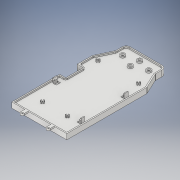
# Autodesk Inventor part: Display_Plate
Saved by Autodesk Inventor 2018 (Build 220112000, 112)
## iProperties
Created: 2019-05-28
Part Number: Display_Plate
Material: ABS Plastic
Document SubType Name: Modeling
Designer: Ash
Density: 1.06 g/cm^3
Appearance: Smooth - White
Author: Ash
Autodesk Inventor part; units mm, degrees
ref_plane "YZ Plane" through (0, 0, 0) normal (1, 0, 0) x (0, 1, 0)
ref_plane "XZ Plane" through (0, 0, 0) normal (0, 1, 0) x (-1, 0, 0)
ref_plane "XY Plane" through (0, 0, 0) normal (0, 0, 1) x (1, 0, 0)
sketch "Sketch1" plane through (0, 0, 0) normal (0, 1, 0) x (-1, 0, 0)
  line L0 (-80.01, -1.2579) -> (-80.01, -117.3941)
  line L1 (-80.01, -118.0979) -> (0, -118.0979) construction
  line L2 (0, -117.3941) -> (0, -96.3809)
  line L3 (-79.7125, -118.7359) -> (-69.5125, -140.61)
  line L4 (-80.01, -118.0979) -> (-55.8746, -118.0979) construction
  line L5 (-0.2975, -118.7359) -> (-10.4975, -140.61)
  line L6 (0, -118.0979) -> (24.1354, -118.0979) construction
  line L7 (-10.795, -141.2479) -> (-69.215, -141.2479) construction
  line L8 (-69.215, -141.9518) -> (-69.215, -150.6459)
  line L9 (-62.865, -156.9959) -> (-17.145, -156.9959)
  line L10 (-10.795, -150.6459) -> (-10.795, -141.9518)
  arc A0 (-0.2975, -118.7359) -> (0, -117.3941) centre (-3.175, -117.3941) ccw
  arc A1 (-80.01, -117.3941) -> (-79.7125, -118.7359) centre (-76.835, -117.3941) ccw
  arc A2 (-69.215, -150.6459) -> (-62.865, -156.9959) centre (-62.865, -150.6459) ccw
  arc A3 (-17.145, -156.9959) -> (-10.795, -150.6459) centre (-17.145, -150.6459) ccw
  arc A4 (-10.4975, -140.61) -> (-10.795, -141.9518) centre (-7.62, -141.9518) ccw
  arc A5 (-69.215, -141.9518) -> (-69.5125, -140.61) centre (-72.39, -141.9518) ccw
  line L11 (0, -96.3809) -> (-8.763, -96.3809)
  line L12 (-8.763, -96.3809) -> (-8.763, -70.9809)
  line L13 (-8.763, -70.9809) -> (0, -70.9809)
  line L14 (-80.01, -1.2579) -> (0, -1.2579)
  line L15 (0, -70.9809) -> (0, -1.2579)
  point P0 (0, 0)
  point P1 (-69.215, -156.9959)
  dimension "d0" = 80.01
  dimension "d1" = 116.84
  dimension "d3" = 65
  dimension "d4" = 115
  dimension "d5" = 58.42
  dimension "d6" = 15.748
  dimension "d7" = 3.175
  dimension "d8" = 6.35
  dimension "d9" = 3.175
  dimension "d45" = 8.763
  dimension "d46" = 25.4
  dimension "d47" = 21.717
  constraints: 32 end point, 12 point on circle, 12 point on line, 12 tangent, 6 centre point, 5 horizontal, 4 parallel, 4 perpendicular, 3 equal radius, 2 equal length, 1 horizontal alignment, 1 vertical
  measures "d0" distance of L1.end L1.start
  measures "d1" distance of L0.start L1.start
  measures "d3" angle of L3 L4
  measures "d4" angle of L5 L6
  measures "d5" distance of point (-69.215, -141.248) L7.start
  measures "d6" distance of point (-69.215, -156.996) L7.end
  measures "d7" radius of A0
  measures "d8" radius of A2
  measures "d9" radius of A4
  measures "d45" distance of L2.end L11.end
  measures "d46" distance of L11.end L12.end
  measures "d47" distance from line of L1.end L11
extrude "Extrusion1" add sketch "Sketch1" along normal blind 3.81
shell "Shell1" thickness 1.778 removed faces 1 at (56.261, 3.81, -63.211)
sketch "Sketch2" plane through (1.778, 1.778, -1.778) normal (0, 1, 0) x (1, 0, 0)
  arc A0 (65.659, 140.1738) -> (66.1231, 138.0805) centre (70.612, 140.1738) ccw projected
  line L0 (65.7764, 139.1017) -> (60.579, 139.1017)
  line L1 (65.659, 148.8679) -> (65.659, 140.1738) projected
  line L2 (65.659, 140.6257) -> (60.579, 140.6257)
  line L3 (76.454, 115.6161) -> (76.454, 1.2579) projected
  arc A1 (76.454, 115.6161) -> (76.3231, 116.2065) centre (75.057, 115.6161) ccw projected
  line L4 (66.1231, 138.0805) -> (76.3231, 116.2065) projected
  arc A2 (65.659, 140.1738) -> (66.1231, 138.0805) centre (70.612, 140.1738) ccw projected
  line L5 (65.659, 148.8679) -> (65.659, 140.1738) projected
  arc A3 (65.659, 148.8679) -> (61.087, 153.4399) centre (61.087, 148.8679) ccw construction
  line L6 (15.367, 153.4399) -> (61.087, 153.4399) construction
  arc A4 (15.367, 153.4399) -> (10.795, 148.8679) centre (15.367, 148.8679) ccw construction
  line L7 (10.795, 140.1738) -> (10.795, 148.8679) projected
  arc A5 (10.3309, 138.0805) -> (10.795, 140.1738) centre (5.842, 140.1738) ccw projected
  line L8 (0.1309, 116.2065) -> (10.3309, 138.0805) construction
  arc A6 (0.1309, 116.2065) -> (0, 115.6161) centre (1.397, 115.6161) ccw projected
  line L9 (0, 96.3809) -> (0, 115.6161) projected
  circle A7 centre (57.2357, 139.8637) radius 1.905
  circle A8 centre (57.2357, 139.8637) radius 3.429
  line L10 (65.7764, 139.8637) -> (47.2298, 139.8637) construction
  line L11 (15.367, 153.4399) -> (61.087, 153.4399) construction
  line L12 (38.227, 153.4399) -> (38.227, -24.5514) construction
  line L13 (57.2357, 139.8637) -> (57.2357, 153.4399) construction
  line L14 (56.4737, 143.207) -> (56.4737, 153.4399)
  line L15 (57.9977, 143.2111) -> (57.9977, 153.4399)
  line L16 (57.2357, 139.8637) -> (38.227, 145.4827) construction
  line L17 (57.2357, 139.8637) -> (38.227, 132.0207) construction
  circle A9 centre (38.227, 132.0207) radius 1.905
  circle A10 centre (38.227, 145.4827) radius 1.905
  circle A11 centre (38.227, 132.0207) radius 3.429
  circle A12 centre (38.227, 145.4827) radius 3.429
  line L18 (41.6491, 145.2657) -> (54.2456, 141.5422)
  line L19 (59.5161, 139.9683) -> (54.4955, 137.8025) construction
  line L20 (41.2171, 143.8042) -> (53.8136, 140.0807)
  line L21 (54.9501, 139.7414) -> (53.8727, 139.1943) construction
  line L22 (53.8136, 140.0807) -> (54.9501, 139.7414) construction
  line L23 (53.8727, 139.1943) -> (41.0645, 133.946)
  line L24 (54.2456, 141.5422) -> (59.5161, 139.9683) construction
  line L25 (54.4955, 137.8025) -> (41.6186, 132.5261)
  line L26 (10.6776, 139.1017) -> (15.875, 139.1017)
  line L27 (10.795, 140.6257) -> (15.875, 140.6257)
  circle A13 centre (19.2183, 139.8637) radius 1.905
  circle A14 centre (19.2183, 139.8637) radius 3.429
  line L28 (19.9803, 143.207) -> (19.9803, 153.4399)
  line L29 (18.4563, 143.2111) -> (18.4563, 153.4399)
  line L30 (34.8049, 145.2657) -> (22.2084, 141.5422)
  line L31 (35.2369, 143.8042) -> (22.6404, 140.0807)
  line L32 (22.5813, 139.1943) -> (35.3895, 133.946)
  line L33 (21.9585, 137.8025) -> (34.8354, 132.5261)
  line L34 (34.8354, 132.5261) -> (21.9585, 137.8025)
  line L35 (22.5813, 139.1943) -> (35.3895, 133.946)
  circle A15 centre (38.227, 132.0207) radius 3.429
  circle A16 centre (38.227, 145.4827) radius 3.429
  circle A17 centre (19.2183, 139.8637) radius 3.429
  line L36 (15.367, 153.4399) -> (61.087, 153.4399) projected
  line L37 (8.763, 96.3809) -> (0, 96.3809) projected
  line L38 (8.763, 67.4249) -> (8.763, 96.3809) projected
  line L39 (0, 67.4249) -> (8.763, 67.4249) projected
  line L40 (0, 1.2579) -> (0, 67.4249) projected
  line L41 (76.454, 1.2579) -> (0, 1.2579) projected
  point P0 (-1.778, -1.778)
  dimension "d13" = 1.524
  dimension "d14" = 5.08
  dimension "d15" = 3.81
  dimension "d16" = 1.524
  dimension "d17" = 0.762
  dimension "d20" = 1.524
  dimension "d21" = 0.762
  dimension "d22" = 13.462
  dimension "d23" = 3.81
  dimension "d24" = 3.81
  dimension "d25" = 1.524
  dimension "d26" = 1.524
  dimension "d27" = 0.762
  dimension "d28" = 0.762
  dimension "d30" = 1.524
  constraints: 54 end point, 17 symmetric about line, 7 centre point, 7 point on line, 6 point on circle, 5 coincident, 4 parallel, 2 horizontal, 2 vertical, 1 concentric, 1 midpoint, 1 perpendicular, 28 other
  measures "d13" distance between parallel lines of L0 L2
  measures "d14" distance of L2.start L2.end
  measures "d15" diameter of A7
  measures "d17" distance between parallel lines of L0 L10
  measures "d20" distance between parallel lines of L15 L14
  measures "d21" distance between parallel lines of L13 L14
  measures "d22" distance of L16.end L17.end
  measures "d23" diameter of A9
  measures "d24" diameter of A10
  measures "d25" radial gap between concentric circles of A9 A11
  measures "d26" radial gap between concentric circles of A10 A12
  measures "d27" distance between parallel lines of L16 L18
  measures "d28" distance between parallel lines of L16 L20
  measures "d30" distance between parallel lines of L25 L23
sketch "Sketch3" plane through (1.778, 1.778, -1.778) normal (0, 1, 0) x (1, 0, 0)
  circle A0 centre (19.2183, 139.7488) radius 1.905 projected
  circle A1 centre (19.2183, 139.7488) radius 3.429 projected
  circle A2 centre (38.227, 145.4827) radius 1.905 projected
  circle A3 centre (38.227, 145.4827) radius 3.429 projected
  circle A4 centre (38.227, 132.0207) radius 1.905 projected
  circle A5 centre (38.227, 132.0207) radius 3.429 projected
  circle A6 centre (57.2357, 139.7488) radius 1.905 projected
  circle A7 centre (57.2357, 139.7488) radius 3.429 projected
  arc A8 (60.579, 140.5108) -> (60.579, 140.5108) centre (57.2357, 139.7488) ccw projected
  line L0 (58.0015, 143.0912) -> (58.0015, 153.325)
  line L1 (15.367, 153.4399) -> (61.087, 153.4399) projected
  line L2 (56.4718, 153.325) -> (56.4718, 143.0916)
  line L3 (65.659, 148.8679) -> (65.659, 140.1738) projected
  arc A9 (65.659, 148.8679) -> (61.087, 153.4399) centre (61.087, 148.8679) ccw projected
  line L4 (15.367, 153.4399) -> (61.087, 153.4399) projected
  arc A10 (15.367, 153.4399) -> (10.795, 148.8679) centre (15.367, 148.8679) ccw projected
  line L5 (10.795, 140.1738) -> (10.795, 148.8679) projected
  arc A11 (10.3309, 138.0805) -> (10.795, 140.1738) centre (5.842, 140.1738) ccw projected
  line L6 (0.1309, 116.2065) -> (10.3309, 138.0805) projected
  arc A12 (0.1309, 116.2065) -> (0, 115.6161) centre (1.397, 115.6161) ccw projected
  line L7 (0, 96.3809) -> (0, 115.6161) projected
  line L8 (76.454, 115.6161) -> (76.454, 1.2579) projected
  arc A13 (76.454, 115.6161) -> (76.3231, 116.2065) centre (75.057, 115.6161) ccw projected
  line L9 (66.1231, 138.0805) -> (76.3231, 116.2065) projected
  arc A14 (65.659, 140.1738) -> (66.1231, 138.0805) centre (70.612, 140.1738) ccw projected
  line L10 (18.4767, 153.4399) -> (18.4767, 143.2116)
  circle A15 centre (19.2183, 139.7488) radius 3.429 projected
  line L11 (19.9598, 143.0967) -> (19.9598, 153.4399)
  line L12 (22.199, 141.4439) -> (34.8061, 145.2467)
  arc A16 (41.656, 145.4827) -> (41.656, 145.4827) centre (38.227, 145.4827) ccw projected
  line L13 (35.2463, 143.7877) -> (22.6391, 139.9848)
  line L14 (22.023, 137.7761) -> (34.8354, 132.5261)
  arc A17 (41.656, 132.0207) -> (41.656, 132.0207) centre (38.227, 132.0207) ccw projected
  line L15 (22.6008, 139.1863) -> (35.3895, 133.946)
  line L16 (15.875, 140.5108) -> (10.795, 140.5108)
  line L17 (10.795, 140.1738) -> (10.795, 148.8679) projected
  line L18 (15.875, 138.9868) -> (10.6776, 139.1017)
  line L19 (8.763, 96.3809) -> (0, 96.3809) projected
  line L20 (8.763, 67.4249) -> (8.763, 96.3809) projected
  line L21 (0, 67.4249) -> (8.763, 67.4249) projected
  line L22 (0, 1.2579) -> (0, 67.4249) projected
  line L23 (76.454, 1.2579) -> (0, 1.2579) projected
  point P0 (-1.778, -1.778)
  constraints: 20 end point, 7 point on circle, 3 point on line, 2 parallel, 2 vertical, 1 horizontal, 1 perpendicular, 9 other
sketch "Sketch5" plane through (1.778, 1.778, -1.778) normal (0, 1, 0) x (1, 0, 0)
  line L0 (0, 96.3809) -> (0, 115.6161) projected
  line L1 (0, 115.6161) -> (10.16, 115.6161) construction
  arc A0 (76.454, 115.6161) -> (76.3231, 116.2065) centre (75.057, 115.6161) ccw projected
  line L2 (76.3231, 116.2065) -> (66.1631, 116.2065) construction
  line L3 (-1.778, 69.2029) -> (-1.778, -1.778) projected
  line L4 (-1.778, 23.1379) -> (19.304, 23.1379) construction
  line L5 (-1.778, 23.1379) -> (19.304, 23.1379) construction
  line L6 (76.454, 23.1379) -> (55.372, 23.1379) construction
  line L7 (61.087, 155.2179) -> (15.367, 155.2179) projected
  line L8 (9.4963, 155.2179) -> (45.0563, 155.2179) construction
  line L9 (10.795, 140.5108) -> (22.6473, 140.5108) construction
  line L10 (10.16, 116.3781) -> (5.08, 116.3781)
  line L11 (5.08, 116.3781) -> (5.08, 114.8541)
  line L12 (5.08, 114.8541) -> (10.16, 114.8541)
  line L13 (10.16, 114.8541) -> (10.16, 116.3781)
  line L14 (6.858, 113.0761) -> (8.382, 113.0761)
  line L15 (8.382, 113.0761) -> (8.382, 118.1561)
  line L16 (8.382, 118.1561) -> (6.858, 118.1561)
  line L17 (6.858, 118.1561) -> (6.858, 113.0761)
  line L18 (6.858, 113.0761) -> (8.382, 118.1561) construction
  line L19 (8.382, 113.0761) -> (6.858, 118.1561) construction
  line L20 (7.62, 116.3781) -> (7.62, 114.8541) construction
  circle A1 centre (7.62, 115.6161) radius 0.889
  line L21 (68.7031, 115.4445) -> (63.6231, 115.4445)
  line L22 (63.6231, 115.4445) -> (63.6231, 116.9685)
  line L23 (63.6231, 116.9685) -> (68.7031, 116.9685)
  line L24 (68.7031, 116.9685) -> (68.7031, 115.4445)
  line L25 (65.4011, 113.6665) -> (66.9251, 113.6665)
  line L26 (66.9251, 113.6665) -> (66.9251, 118.7465)
  line L27 (66.9251, 118.7465) -> (65.4011, 118.7465)
  line L28 (65.4011, 118.7465) -> (65.4011, 113.6665)
  line L29 (65.4011, 113.6665) -> (66.9251, 118.7465) construction
  line L30 (66.9251, 113.6665) -> (65.4011, 118.7465) construction
  line L31 (66.1631, 115.4445) -> (66.1631, 116.9685) construction
  circle A2 centre (66.1631, 116.2065) radius 0.889
  line L32 (54.61, 20.5979) -> (56.134, 20.5979)
  line L33 (55.372, 22.3759) -> (55.372, 23.8999) construction
  line L34 (52.832, 23.8999) -> (57.912, 23.8999)
  circle A3 centre (55.372, 23.1379) radius 0.889
  line L35 (57.912, 23.8999) -> (57.912, 22.3759)
  line L36 (57.912, 22.3759) -> (52.832, 22.3759)
  line L37 (56.134, 20.5979) -> (56.134, 25.6779)
  line L38 (54.61, 20.5979) -> (56.134, 25.6779) construction
  line L39 (56.134, 20.5979) -> (54.61, 25.6779) construction
  line L40 (54.61, 25.6779) -> (54.61, 20.5979)
  line L41 (56.134, 25.6779) -> (54.61, 25.6779)
  line L42 (52.832, 22.3759) -> (52.832, 23.8999)
  line L43 (18.542, 20.5979) -> (20.066, 20.5979)
  line L44 (19.304, 22.3759) -> (19.304, 23.8999) construction
  line L45 (16.764, 23.8999) -> (21.844, 23.8999)
  circle A4 centre (19.304, 23.1379) radius 0.889
  line L46 (21.844, 23.8999) -> (21.844, 22.3759)
  line L47 (21.844, 22.3759) -> (16.764, 22.3759)
  line L48 (20.066, 20.5979) -> (20.066, 25.6779)
  line L49 (18.542, 20.5979) -> (20.066, 25.6779) construction
  line L50 (20.066, 20.5979) -> (18.542, 25.6779) construction
  line L51 (18.542, 25.6779) -> (18.542, 20.5979)
  line L52 (20.066, 25.6779) -> (18.542, 25.6779)
  line L53 (16.764, 22.3759) -> (16.764, 23.8999)
  line L54 (76.454, 115.6161) -> (76.454, 1.2579) projected
  line L55 (76.454, 0) -> (0, 0) projected
  point P0 (22.6473, 139.7488)
  point P1 (68.7031, 117.2036)
  point P2 (57.912, 118.7911)
  point P3 (55.372, 23.1379)
  point P4 (21.844, 120.3786)
  point P5 (19.304, 23.1379)
  point P6 (7.62, 115.6161)
  dimension "d48" = 10.16
  dimension "d49" = 10.16
  dimension "d50" = 21.082
  dimension "d52" = 21.082
  dimension "d56" = 0.762
  dimension "d57" = 0.762
  dimension "d58" = 5.08
  dimension "d59" = 1.524
  dimension "d60" = 5.08
  dimension "d61" = 1.778
  dimension "d66" = 5.08
  dimension "d67" = 1.524
  dimension "d68" = 5.08
  dimension "d69" = 1.778
  dimension "d70" = 1.524
  dimension "d71" = 5.08
  dimension "d72" = 1.524
  dimension "d73" = 5.08
  dimension "d74" = 1.778
  dimension "d75" = 1.524
  dimension "d76" = 5.08
  dimension "d77" = 1.524
  dimension "d78" = 5.08
  dimension "d79" = 1.778
  dimension "d80" = 1.524
  dimension "d160" = 132.08
  constraints: 100 end point, 27 midpoint, 16 parallel, 12 horizontal, 9 perpendicular, 9 point on line, 4 centre point, 4 coincident, 1 collinear
  measures "d48" distance of L0.end L1.end
  measures "d49" distance of L2.start L2.end
  measures "d50" distance of L4.end L4.start
  measures "d52" distance of L6.end L6.start
  measures "d56" distance between parallel lines of L1 L10
  measures "d57" distance between parallel lines of L1 L12
  measures "d58" distance between parallel lines of L13 L11
  measures "d59" distance of L16.end L15.end
  measures "d60" distance of L15.end L14.end
  measures "d61" diameter of A1
  measures "d66" distance between parallel lines of L24 L22
  measures "d67" distance of L30.end L26.end
  measures "d68" distance of L26.end L25.end
  measures "d69" diameter of A2
  measures "d70" distance between parallel lines of L21 L23
  measures "d71" distance between parallel lines of L35 L42
  measures "d72" distance of L41.end L37.end
  measures "d73" distance of L37.end L32.end
  measures "d74" diameter of A3
  measures "d75" distance between parallel lines of L36 L34
  measures "d76" distance between parallel lines of L46 L53
  measures "d77" distance of L52.end L48.end
  measures "d78" distance of L48.end L43.end
  measures "d79" diameter of A4
  measures "d80" distance between parallel lines of L47 L45
  measures "d160" distance between parallel lines of L7 L6
extrude "Extrusion7" add sketch "Sketch5" along normal blind 3.048 contours A1 L15 L12 L17 L10 | L10 A1 | A1 L15 | A1 L12 | L17 A1 | A2 L21 | L21 A2 L28 L23 L26 | L26 A2 | L23 A2 | A2 L28 | L36 A3 | A3 L40 L34 L37 L36 | A3 L40 | L37 A3 | A3 L34 | L47 A4 | A4 L51 L45 L48 L47 | A4 L51 | L48 A4 | A4 L45
extrude "Extrusion8" add sketch "Sketch5" along normal up to surface (2.032 mm away)
sketch "Sketch6" plane through (1.778, 1.778, -1.778) normal (0, 1, 0) x (1, 0, 0)
  line L0 (3.302, 61.0749) -> (7.366, 61.0749)
  line L1 (7.366, 61.0749) -> (7.366, 54.9789)
  line L2 (7.366, 54.9789) -> (3.302, 54.9789)
  line L3 (3.302, 54.9789) -> (3.302, 61.0749)
  line L4 (0, 67.4249) -> (8.763, 67.4249) projected
  line L5 (6.985, 69.2029) -> (-1.778, 69.2029) projected
  line L6 (-1.778, 69.2029) -> (-1.778, -1.778) projected
  line L7 (69.088, 29.718) -> (73.152, 29.718)
  line L8 (73.152, 29.718) -> (73.152, 23.622)
  line L9 (73.152, 23.622) -> (69.088, 23.622)
  line L10 (69.088, 23.622) -> (69.088, 29.718)
  line L11 (78.232, -0.5201) -> (78.232, 115.6161) projected
  line L12 (-1.778, -1.778) -> (78.232, -1.778) projected
  line L13 (69.088, 93.218) -> (73.152, 93.218)
  line L14 (73.152, 93.218) -> (73.152, 87.122)
  line L15 (73.152, 87.122) -> (69.088, 87.122)
  line L16 (69.088, 87.122) -> (69.088, 93.218)
  line L17 (76.454, 115.6161) -> (76.454, 1.2579) projected
  point P0 (0, 67.31)
  point P1 (76.454, 0)
  dimension "d82" = 4.064
  dimension "d83" = 6.096
  dimension "d85" = 8.128
  dimension "d86" = 5.08
  dimension "d87" = 4.064
  dimension "d88" = 6.096
  dimension "d89" = 5.08
  dimension "d90" = 25.4
  dimension "d91" = 4.064
  dimension "d92" = 6.096
  dimension "d93" = 88.9
  dimension "d95" = 5.08
  constraints: 24 end point, 6 parallel, 3 horizontal, 3 perpendicular, 1 other
  measures "d82" distance of L1.end L2.end
  measures "d83" distance of L0.end L1.end
  measures "d85" distance between parallel lines of L5 L0
  measures "d86" distance between parallel lines of L6 L3
  measures "d87" distance of L8.end L9.end
  measures "d88" distance of L7.end L8.end
  measures "d89" distance between parallel lines of L11 L8
  measures "d90" distance between parallel lines of L12 L9
  measures "d91" distance of L14.end L15.end
  measures "d92" distance of L13.end L14.end
  measures "d93" distance between parallel lines of L12 L15
  measures "d95" distance between parallel lines of L11 L14
extrude "Extrusion9" cut sketch "Sketch6" against normal through all
sketch "Sketch7" plane through (1.778, 1.778, -1.778) normal (0, 1, 0) x (1, 0, 0)
  line L0 (3.302, 54.9789) -> (3.302, 61.0749) projected
  line L1 (3.302, 60.4399) -> (2.032, 60.4399)
  line L2 (2.032, 60.4399) -> (2.032, 55.4869)
  line L3 (2.032, 55.4869) -> (3.302, 55.4869)
  line L4 (3.302, 55.4869) -> (3.302, 60.4399)
  line L5 (3.302, 61.0749) -> (7.366, 61.0749) projected
  line L6 (74.422, 92.583) -> (73.152, 92.583)
  line L7 (73.152, 92.583) -> (73.152, 87.63)
  line L8 (73.152, 87.63) -> (74.422, 87.63)
  line L9 (74.422, 87.63) -> (74.422, 92.583)
  line L10 (73.152, 93.218) -> (73.152, 87.122) projected
  line L11 (69.088, 93.218) -> (73.152, 93.218) projected
  line L12 (74.422, 29.21) -> (73.152, 29.21)
  line L13 (73.152, 29.21) -> (73.152, 24.257)
  line L14 (73.152, 24.257) -> (74.422, 24.257)
  line L15 (74.422, 24.257) -> (74.422, 29.21)
  line L16 (73.152, 29.718) -> (73.152, 23.622) projected
  line L17 (69.088, 29.718) -> (73.152, 29.718) projected
  line L18 (73.152, 23.622) -> (69.088, 23.622) projected
  point P0 (-1.778, -1.778)
  dimension "d98" = 1.27
  dimension "d99" = 4.953
  dimension "d100" = 0.635
  dimension "d103" = 1.27
  dimension "d104" = 4.953
  dimension "d105" = 0.635
  dimension "d106" = 1.27
  dimension "d107" = 4.953
  dimension "d109" = 0.635
  constraints: 24 end point, 6 parallel, 3 horizontal, 3 perpendicular, 2 collinear, 1 point on line
  measures "d98" distance of L3.end L2.end
  measures "d99" distance of L2.end L1.end
  measures "d100" distance between parallel lines of L5 L1
  measures "d103" distance of L8.end L7.end
  measures "d104" distance of L7.end L6.end
  measures "d105" distance between parallel lines of L11 L6
  measures "d106" distance of L14.end L13.end
  measures "d107" distance of L13.end L12.end
  measures "d109" distance between parallel lines of L18 L14
extrude "Extrusion10" add sketch "Sketch7" along normal blind 6.604
sketch "Sketch8" plane through (3.81, 1.778, -57.2649) normal (0, 0, 1) x (1, 0, 0)
  line L0 (1.27, 0) -> (1.27, 6.604) projected
  line L1 (1.27, 6.604) -> (2.286, 4.064)
  line L2 (2.286, 4.064) -> (1.27, 4.064)
  line L3 (0, 0) -> (0, 6.604) projected
  line L4 (0, 6.604) -> (1.27, 6.604) projected
  point P0 (-3.81, -1.778)
  dimension "d111" = 2.286
  dimension "d115" = 2.54
  constraints: 4 end point, 1 perpendicular, 1 point on line
  measures "d111" distance from line of L3 L1.end
  measures "d115" distance between parallel lines of L4 L2
extrude "Extrusion11" add sketch "Sketch8" against normal up to surface (4.953 mm away)
sketch "Sketch10" plane through (74.93, 1.778, -89.408) normal (0, 0, 1) x (1, 0, 0)
  line L0 (0, 0) -> (0, 6.604) projected
  line L1 (0, 6.604) -> (-1.016, 4.064)
  line L2 (-1.016, 4.064) -> (0, 4.064)
  line L3 (1.27, 0) -> (1.27, 6.604) projected
  line L4 (0, 6.604) -> (1.27, 6.604) projected
  point P0 (-74.93, -1.778)
  dimension "d114" = 2.286
  dimension "d116" = 2.54
  constraints: 4 end point, 1 horizontal, 1 point on line
  measures "d114" distance from line of L3 L1.end
  measures "d116" distance between parallel lines of L4 L2
sketch "Sketch11" plane through (74.93, 1.778, -26.035) normal (0, 0, 1) x (1, 0, 0)
  line L0 (0, 0) -> (0, 6.604) projected
  line L1 (0, 6.604) -> (-1.016, 4.064)
  line L2 (-1.016, 4.064) -> (0, 4.064)
  line L3 (1.27, 0) -> (1.27, 6.604) projected
  line L4 (0, 6.604) -> (1.27, 6.604) projected
  point P0 (-74.93, -1.778)
  dimension "d117" = 2.286
  dimension "d118" = 2.54
  constraints: 4 end point, 1 horizontal, 1 point on line
  measures "d117" distance from line of L3 L1.end
  measures "d118" distance between parallel lines of L4 L2
extrude "Extrusion12" add sketch "Sketch11" against normal up to surface (4.953 mm away)
extrude "Extrusion13" add sketch "Sketch10" against normal up to surface (4.953 mm away)
extrude "Extrusion14" cut sketch "Sketch3" against normal through all contours A0 | A2 | A4 | A6
sketch "Sketch12" plane through (0, 0, 0) normal (0, -1, 0) x (1, 0, 0)
  circle A0 centre (40.005, -133.7987) radius 1.905 projected
  circle A1 centre (20.9963, -141.5268) radius 1.905 projected
  circle A2 centre (40.005, -147.2607) radius 1.905 projected
  circle A3 centre (59.0137, -141.5268) radius 1.905 projected
  line L0 (70.866, -31.496) -> (70.866, -25.4) projected
  line L1 (70.866, -25.4) -> (74.93, -25.4) projected
  line L2 (74.93, -25.4) -> (74.93, -31.496) projected
  line L3 (74.93, -31.496) -> (70.866, -31.496) projected
  line L4 (5.08, -62.8529) -> (5.08, -56.7569) projected
  line L5 (5.08, -56.7569) -> (9.144, -56.7569) projected
  line L6 (9.144, -56.7569) -> (9.144, -62.8529) projected
  line L7 (9.144, -62.8529) -> (5.08, -62.8529) projected
  line L8 (70.866, -94.996) -> (70.866, -88.9) projected
  line L9 (70.866, -88.9) -> (74.93, -88.9) projected
  line L10 (74.93, -88.9) -> (74.93, -94.996) projected
  line L11 (74.93, -94.996) -> (70.866, -94.996) projected
  line L12 (0, -70.9809) -> (8.763, -70.9809) projected
  line L13 (8.763, -70.9809) -> (8.763, -96.3809) projected
  line L14 (8.763, -96.3809) -> (0, -96.3809) projected
  line L15 (0, -96.3809) -> (0, -117.3941) projected
  arc A4 (0, -117.3941) -> (0.2975, -118.7359) centre (3.175, -117.3941) ccw projected
  line L16 (0.2975, -118.7359) -> (10.4975, -140.61) projected
  arc A5 (10.795, -141.9518) -> (10.4975, -140.61) centre (7.62, -141.9518) ccw projected
  line L17 (10.795, -141.9518) -> (10.795, -150.6459) projected
  arc A6 (10.795, -150.6459) -> (17.145, -156.9959) centre (17.145, -150.6459) ccw projected
  line L18 (17.145, -156.9959) -> (62.865, -156.9959) projected
  arc A7 (62.865, -156.9959) -> (69.215, -150.6459) centre (62.865, -150.6459) ccw projected
  line L19 (69.215, -150.6459) -> (69.215, -141.9518) projected
  arc A8 (69.5125, -140.61) -> (69.215, -141.9518) centre (72.39, -141.9518) ccw projected
  line L20 (69.5125, -140.61) -> (79.7125, -118.7359) projected
  arc A9 (79.7125, -118.7359) -> (80.01, -117.3941) centre (76.835, -117.3941) ccw projected
  line L21 (80.01, -117.3941) -> (80.01, -1.2579) projected
  arc A10 (62.865, -155.7259) -> (67.945, -150.6459) centre (62.865, -150.6459) ccw
  line L22 (62.865, -155.7259) -> (17.145, -155.7259)
  arc A11 (12.065, -150.6459) -> (17.145, -155.7259) centre (17.145, -150.6459) ccw
  line L23 (12.065, -150.6459) -> (12.065, -141.9518)
  arc A12 (1.27, -117.3941) -> (1.4485, -118.1991) centre (3.175, -117.3941) ccw
  line L24 (1.27, -117.3941) -> (1.27, -97.6509)
  line L25 (1.27, -97.6509) -> (10.033, -97.6509)
  line L26 (10.033, -97.6509) -> (10.033, -69.7109)
  line L27 (10.033, -69.7109) -> (1.27, -69.7109)
  line L28 (1.27, -69.7109) -> (1.27, -1.3849)
  line L29 (1.27, -1.3849) -> (78.74, -1.3849)
  line L30 (78.74, -1.3849) -> (78.74, -117.3941)
  arc A13 (78.5615, -118.1991) -> (78.74, -117.3941) centre (76.835, -117.3941) ccw
  line L31 (78.5615, -118.1991) -> (69.215, -138.2428)
  line L32 (67.945, -141.9518) -> (67.945, -150.6459)
  line L33 (67.5544, -140.7648) -> (62.357, -140.7648) projected
  line L34 (67.945, -141.9518) -> (12.065, -141.9518) construction
  arc A14 (67.945, -133.2577) -> (62.865, -128.1777) centre (62.865, -133.2577) ccw
  line L35 (62.865, -128.1777) -> (17.145, -128.1777)
  arc A15 (17.145, -128.1777) -> (12.065, -133.2577) centre (17.145, -133.2577) ccw
  line L36 (12.065, -133.2577) -> (12.065, -141.9518)
  line L37 (67.945, -141.9518) -> (67.945, -133.2577)
  line L38 (10.795, -133.2577) -> (10.795, -141.9518)
  arc A16 (17.145, -126.9077) -> (10.795, -133.2577) centre (17.145, -133.2577) ccw
  line L39 (62.865, -126.9077) -> (17.145, -126.9077)
  arc A17 (69.215, -133.2577) -> (62.865, -126.9077) centre (62.865, -133.2577) ccw
  line L40 (69.215, -141.9518) -> (69.215, -133.2577)
  line L41 (10.795, -138.2428) -> (1.4485, -118.1991)
  line L42 (80.01, -1.2579) -> (0, -1.2579) projected
  line L43 (0, -1.2579) -> (0, -70.9809) projected
  point P0 (0, 0)
  point P1 (67.437, -142.2888)
  dimension "d125" = 1.27
  constraints: 38 end point, 16 point on circle, 12 symmetric about line, 8 centre point, 2 point on line, 12 other
  measures "d125" radial gap between concentric circles of A7 A10
extrude "Extrusion15" add sketch "Sketch12" along normal blind 4.064 contours L0 L1 L2 L3 | L4 L5 L6 L7 | L8 L9 L10 L11 | L43 L42 L21 A9 L20 A8 L40 L31 A13 L30 L29 L28 L27 L26 L25 L24 A12 L41 L38 A5 L16 A4 L15 L14 L13 L12 | L40 A17 L39 A16 L38 L41 A12 L24 L25 L26 L27 L28 L29 L30 A13 L31
sketch "Sketch13" plane through (0, 0, 0) normal (0, -1, 0) x (1, 0, 0)
  line L0 (76.2, -7.366) -> (9.144, -7.366)
  line L1 (9.144, -7.366) -> (9.144, -113.03)
  line L2 (9.144, -113.03) -> (76.2, -113.03)
  line L3 (76.2, -113.03) -> (76.2, -7.366)
  line L4 (0, 0) -> (80.01, 0) projected
  line L5 (80.01, -117.3941) -> (80.01, -1.2579) projected
  line L6 (77.724, -5.842) -> (7.62, -5.842)
  line L7 (7.62, -5.842) -> (7.62, -114.554)
  line L8 (7.62, -114.554) -> (77.724, -114.554)
  line L9 (77.724, -114.554) -> (77.724, -5.842)
  line L10 (77.724, -21.082) -> (76.2, -21.082)
  line L11 (70.104, -7.366) -> (70.104, -5.842)
  line L12 (9.144, -21.082) -> (7.62, -21.082)
  line L13 (15.24, -7.366) -> (15.24, -5.842)
  line L14 (77.724, -99.314) -> (76.2, -99.314)
  line L15 (70.104, -113.03) -> (70.104, -114.554)
  line L16 (15.24, -114.554) -> (15.24, -113.03)
  line L17 (9.144, -99.314) -> (7.62, -99.314)
  dimension "d128" = 67.056
  dimension "d129" = 105.664
  dimension "d130" = 7.366
  dimension "d131" = 3.81
  dimension "d132" = 1.524
  dimension "d133" = 15.24
  dimension "d134" = 7.62
  dimension "d135" = 7.62
  dimension "d136" = 15.24
  dimension "d137" = 15.24
  dimension "d138" = 7.62
  dimension "d139" = 15.24
  dimension "d140" = 7.62
  constraints: 32 end point, 16 point on line, 9 perpendicular, 5 parallel, 1 horizontal, 3 other
  measures "d128" distance of L2.end L1.end
  measures "d129" distance of L1.end L0.end
  measures "d130" distance between parallel lines of L4 L0
  measures "d131" distance between parallel lines of L5 L3
  measures "d132" distance between parallel lines of L3 L9
  measures "d133" distance between parallel lines of L6 L10
  measures "d134" distance between parallel lines of L9 L11
  measures "d135" distance between parallel lines of L7 L13
  measures "d136" distance between parallel lines of L6 L12
  measures "d137" distance between parallel lines of L8 L17
  measures "d138" distance between parallel lines of L7 L16
  measures "d139" distance between parallel lines of L8 L14
  measures "d140" distance between parallel lines of L9 L15
extrude "Extrusion16" add sketch "Sketch13" along normal blind 3.048 contours L0 L11 L6 L9 L10 L3 | L0 L1 L12 L7 L6 L13 | L14 L9 L8 L15 L2 L3 | L1 L2 L16 L8 L7 L17
fillet "Fillet1" radius 0.8458 4 edges at (56.261, 4.826, -24.9159) (20.193, 4.826, -24.9159) (8.509, 4.826, -117.3941) (67.0521, 4.826, -117.9845)
sketch "Sketch14" plane through (0, 3.81, 0) normal (0, 1, 0) x (1, 0, 0)
  circle A0 centre (21.209, -4.4063) radius 2.413
  line L0 (23.622, -4.4063) -> (23.622, 1.2579)
  line L1 (18.796, -4.4063) -> (18.796, 1.2579)
  circle A1 centre (21.209, -4.4063) radius 0.9525
  circle A2 centre (59.055, -4.4063) radius 2.413
  circle A3 centre (59.055, -4.4063) radius 0.9525
  line L2 (61.468, -4.4063) -> (61.468, 1.2579)
  line L3 (56.642, -4.4063) -> (56.642, 1.2579)
  line L4 (80.01, 1.2579) -> (80.01, 117.3941) projected
  line L5 (0, 1.2579) -> (80.01, 1.2579) projected
  line L6 (0, 70.9809) -> (0, 1.2579) projected
  dimension "d144" = 4.826
  dimension "d146" = 1.905
  dimension "d148" = 4.826
  dimension "d151" = 4.826
  dimension "d152" = 1.905
  dimension "d153" = 4.826
  dimension "d154" = 18.542
  dimension "d163" = 21.209
  dimension "d164" = 5.6642
  constraints: 8 end point, 4 centre point, 4 point on circle, 4 point on line, 3 parallel, 2 coincident, 2 vertical
  measures "d144" diameter of A0
  measures "d146" diameter of A1
  measures "d148" distance between parallel lines of L0 L1
  measures "d151" diameter of A2
  measures "d152" diameter of A3
  measures "d153" distance between parallel lines of L2 L3
  measures "d154" distance between parallel lines of L4 L2
  measures "d163" distance from line of L6 A0.centre
  measures "d164" distance from line of L5 A3.centre
extrude "Extrusion17" add sketch "Sketch14" against normal blind 2.286
fillet "Fillet2" radius 3.175 2 edges at (10.541, 2.794, -69.2029) (10.541, 2.794, -98.1589)
fillet "Fillet3" radius 3.175 1 edges at (1.778, 2.794, -98.1589)
extrude "Extrusion18" add sketch "Sketch2" along normal up to surface (2.032 mm away) contours A8 | A11 | A12 | A14
sketch "Sketch15" plane through (0, 0, 0) normal (0, -1, 0) x (1, 0, 0)
  line L0 (10.795, -133.2577) -> (10.795, -141.9518) projected
  line L1 (10.795, -141.9518) -> (10.795, -150.6459) projected
  arc A0 (10.795, -150.6459) -> (17.145, -156.9959) centre (17.145, -150.6459) ccw projected
  line L2 (17.145, -156.9959) -> (62.865, -156.9959) projected
  arc A1 (62.865, -156.9959) -> (69.215, -150.6459) centre (62.865, -150.6459) ccw projected
  line L3 (69.215, -150.6459) -> (69.215, -141.9518) projected
  line L4 (69.215, -141.9518) -> (69.215, -133.2577) projected
  arc A2 (69.215, -133.2577) -> (62.865, -126.9077) centre (62.865, -133.2577) ccw projected
  line L5 (62.865, -126.9077) -> (17.145, -126.9077) projected
  arc A3 (17.145, -126.9077) -> (10.795, -133.2577) centre (17.145, -133.2577) ccw projected
  circle A4 centre (40.005, -133.7987) radius 1.905 projected
  circle A5 centre (20.9963, -141.5268) radius 1.905 projected
  circle A6 centre (40.005, -147.2607) radius 1.905 projected
  circle A7 centre (59.0137, -141.5268) radius 1.905 projected
  line L6 (17.145, -128.4317) -> (62.865, -128.4317)
  arc A8 (67.691, -133.2577) -> (62.865, -128.4317) centre (62.865, -133.2577) ccw
  line L7 (67.691, -133.2577) -> (67.691, -141.9518)
  line L8 (67.691, -141.9518) -> (67.691, -150.6459)
  arc A9 (62.865, -155.4719) -> (67.691, -150.6459) centre (62.865, -150.6459) ccw
  line L9 (62.865, -155.4719) -> (17.145, -155.4719)
  arc A10 (12.319, -150.6459) -> (17.145, -155.4719) centre (17.145, -150.6459) ccw
  line L10 (12.319, -150.6459) -> (12.319, -141.9518)
  line L11 (12.319, -141.9518) -> (12.319, -133.2577)
  arc A11 (17.145, -128.4317) -> (12.319, -133.2577) centre (17.145, -133.2577) ccw
  point P0 (0, 0)
  dimension "d165" = 1.524
  constraints: 12 end point, 8 point on circle, 4 centre point, 9 other
  measures "d165" distance between parallel lines of L5 L6
extrude "Extrusion19" add sketch "Sketch15" along normal blind 4.572 contours A3 L5 A2 L4 L3 A1 L2 A0 L1 L0
body "Solid1"
